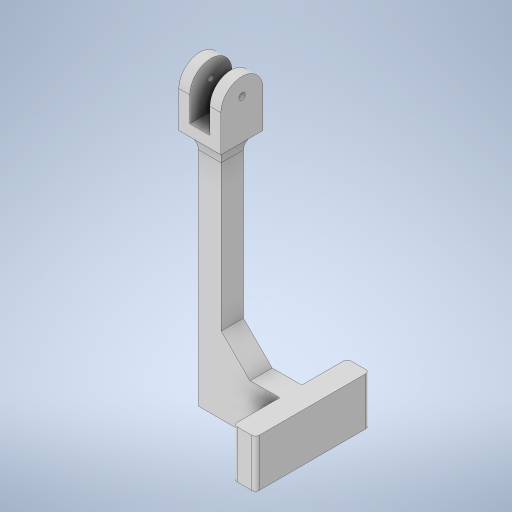
# Autodesk Inventor part: support
Saved by Autodesk Inventor 2023 (Build 270158000, 158)
## iProperties
Created: 2024-05-17
Part Number: support
Material: 一般
Document SubType Name: Modeling
Designer: cadlab
Density: 1 g/cm^3
Appearance: 預設
Author: cadlab
Autodesk Inventor part; units mm, degrees
ref_plane "YZ Plane" through (0, 0, 0) normal (1, 0, 0) x (0, 1, 0)
ref_plane "XZ Plane" through (0, 0, 0) normal (0, 1, 0) x (-1, 0, 0)
ref_plane "XY Plane" through (0, 0, 0) normal (0, 0, 1) x (1, 0, 0)
sketch "草圖1" plane through (0, 0, 0) normal (1, 0, 0) x (0, 1, 0)
  line L0 (6, 5.8) -> (-6, 5.8)
  line L1 (-6, 5.8) -> (-6, -5.8)
  line L2 (-6, -5.8) -> (6, -5.8)
  line L3 (6, -5.8) -> (6, 5.8)
  line L4 (6, 5.8) -> (-6, -5.8) construction
  line L5 (-6, 5.8) -> (6, -5.8) construction
  point P0 (0, 0)
  dimension "d2" = 12
  dimension "d3" = 11.6
  constraints: 12 end point, 2 midpoint, 2 parallel, 1 horizontal, 1 perpendicular
  measures "d2" distance of L1.end L2.end
  measures "d3" distance of L0.end L1.end
extrude "擠出1" add sketch "草圖1" along normal blind 125
sketch "草圖2" plane through (0, 6, 5.8) normal (0, 1, 0) x (1, 0, 0)
  line L0 (0, 0) -> (125, 0) projected
  line L1 (0, 11.6) -> (125, 11.6) projected
  line L2 (0, 0) -> (25, 0)
  line L3 (25, 0) -> (25, 11.6)
  line L4 (25, 11.6) -> (0, 11.6)
  line L5 (0, 11.6) -> (0, 0)
  point P0 (0, 5.8)
  point P1 (0, 11.6)
  dimension "d6" = 25
  constraints: 8 end point, 2 parallel, 1 horizontal, 1 perpendicular, 1 point on line
  measures "d6" distance between parallel lines of L5 L3
extrude "擠出2" add sketch "草圖2" along normal blind 30.5
sketch "草圖3" plane through (0, 36.5, 5.8) normal (0, 1, 0) x (1, 0, 0)
  line L0 (25, 35.8) -> (0, 35.8)
  line L1 (0, 35.8) -> (0, -23.8)
  line L2 (0, -23.8) -> (25, -23.8)
  line L3 (25, -23.8) -> (25, 35.8)
  line L4 (25, 0) -> (25, 11.6) projected
  line L5 (25, 0) -> (125, 0) projected
  point P0 (0, 5.8)
  point P1 (25, 5.8)
  dimension "d9" = 25
  dimension "d10" = 59.6
  dimension "d11" = 23.8
  constraints: 8 end point, 2 parallel, 1 horizontal, 1 midpoint, 1 perpendicular, 1 point on line
  measures "d9" distance between parallel lines of L3 L1
  measures "d10" distance between parallel lines of L2 L0
  measures "d11" distance between parallel lines of L2 L5
extrude "擠出3" add sketch "草圖3" along normal blind 11.6
sketch "草圖4" plane through (125, 0, 0) normal (1, 0, 0) x (0, 0, -1)
  line L0 (-11, -11) -> (11, -11)
  line L1 (11, -11) -> (11, 11)
  line L2 (11, 11) -> (-11, 11)
  line L3 (-11, 11) -> (-11, -11)
  line L4 (-11, -11) -> (11, 11) construction
  line L5 (11, -11) -> (-11, 11) construction
  point P0 (0, 0)
  dimension "d14" = 22
  dimension "d15" = 22
  constraints: 12 end point, 2 midpoint, 2 parallel, 1 horizontal, 1 perpendicular
  measures "d14" distance of L2.end L0.start
  measures "d15" distance of L0.start L0.end
extrude "擠出4" add sketch "草圖4" along normal blind 30
sketch "草圖5" plane through (125, -11, -11) normal (0, 0, -1) x (-1, 0, 0)
  line L0 (-30, 0) -> (-30, 22) projected
  line L1 (-30, 5.75) -> (-6, 5.75)
  line L2 (-6, 5.75) -> (-6, 16.25)
  line L3 (-6, 16.25) -> (-30, 16.25)
  line L4 (-30, 16.25) -> (-30, 5.75)
  line L5 (0, 17) -> (0, 5) projected
  line L6 (0, 11) -> (-32.9331, 11) construction
  point P0 (125, 11)
  dimension "d18" = 10.5
  dimension "d19" = 24
  constraints: 10 end point, 2 horizontal, 2 parallel, 1 midpoint, 1 perpendicular, 1 point on line, 1 other
  measures "d18" distance of L1.end L2.end
  measures "d19" distance of L2.end L3.end
extrude "擠出5" cut sketch "草圖5" against normal blind 30
sketch "草圖6" plane through (125, 11, 11) normal (0, 1, 0) x (1, 0, 0)
  line L0 (6, 22) -> (6, 0) construction
  line L1 (6, 22) -> (6, 0) construction
  line L2 (6, 11) -> (33.0459, 11) construction
  circle A0 centre (21, 11) radius 1.6
  point P0 (-125, 11)
  dimension "d22" = 15
  dimension "d23" = 3.2
  constraints: 2 end point, 1 centre point, 1 horizontal, 1 midpoint, 1 point on line
  measures "d22" distance from line of L0 A0.centre
  measures "d23" diameter of A0
extrude "擠出6" cut sketch "草圖6" against normal blind 30
fillet "圓角1" radius 11 4 edges at (155, 8.125, -11) (155, 8.125, 11) (155, -8.125, 11) (155, -8.125, -11)
fillet "圓角2" radius 10 4 edges at (125, 6, 0) (125, 0, 5.8) (125, 0, -5.8) (125, -6, 0)
chamfer "倒角1" distance 15 angle 45 1 edges at (25, 6, 0)
fillet "圓角3" radius 2 4 edges at (12.5, 48.1, -30) (12.5, 36.5, -30) (12.5, 36.5, 29.6) (12.5, 48.1, 29.6)
